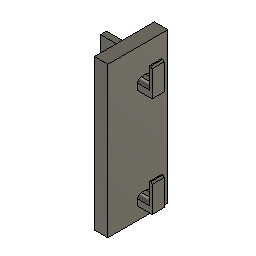
skadis_bracket_right (Autodesk Fusion 360 design; units mm, degrees)
part number: 2026-09-05-18-11-34-603
Autodesk Fusion 360 part; units mm, degrees
sketch "Plate" plane through (0, 0, 0) normal (0, 1, 0) x (1, 0, 0)
  line L0 (0, 0) -> (5.4, 0)
  line L1 (5.4, 0) -> (5.4, -60)
  line L2 (5.4, -60) -> (0, -60)
  line L3 (0, -60) -> (0, 0)
  dimension "d29" = 5.4
  dimension "d30" = 60
  constraint coincident L0.start L3.end
  constraint horizontal L0
  constraint horizontal L2
  constraint vertical L1
  constraint vertical L3
  measures "d29" horizontal distance of L0.start L1.end
  measures "d30" vertical distance of L0.start L1.end
extrude "Plate (1)" add sketch "Plate" along normal mid plane 24
sketch "Hook profile" plane through (0, 0, 0) normal (0, 1, 0) x (1, 0, 0)
  line L0 (0, -58) -> (-8.3, -58)
  line L1 (-8.3, -58) -> (-8.3, -41)
  line L2 (-8.3, -41) -> (-5.3, -41)
  line L3 (-5.3, -41) -> (-3.8, -42.5)
  line L4 (-3.8, -42.5) -> (-3.8, -53)
  line L5 (-3.8, -53) -> (0, -53)
  line L6 (0, -53) -> (0, -58)
  dimension "d33" = 58
  dimension "d34" = 8.3
  dimension "d35" = 3.8
  dimension "d36" = 5
  dimension "d37" = 10.5
  dimension "d38" = 1.5
  dimension "d39" = 1.5
  constraint horizontal L0
  constraint horizontal L2
  constraint horizontal L5
  constraint vertical L1
  constraint vertical L4
  constraint vertical L6
  constraint coincident origin L6
  measures "d33" vertical distance of origin L0.start
  measures "d34" horizontal distance of L0.start L0.end
  measures "d35" horizontal distance of L4.end L5.end
  measures "d36" vertical distance of L0.start L5.end
  measures "d37" vertical distance of L3.end L4.end
  measures "d38" horizontal distance of L2.end L3.end
  measures "d39" vertical distance of L2.end L3.end
extrude "Hook profile (1)" add sketch "Hook profile" along normal mid plane 2.4
pattern_linear "Hook rows" count 2 spacing 25.4 along (0, 0, -1) count 3 spacing 0 along (0, 0, 1) of "Hook profile (1)"
sketch "Peg profile" plane through (0, 0, 0) normal (0, 1, 0) x (1, 0, 0)
  line L0 (5.4, -45) -> (11.2, -45)
  line L1 (11.2, -45) -> (11.2, -55.4)
  line L2 (11.2, -55.4) -> (10.6, -56)
  line L3 (10.6, -56) -> (10.2, -56)
  line L4 (10.2, -56) -> (10.2, -49)
  line L5 (10.2, -49) -> (5.4, -49)
  line L6 (5.4, -49) -> (5.4, -45)
  dimension "d46" = 5.4
  dimension "d47" = 45
  dimension "d48" = 11.2
  dimension "d49" = 55.4
  dimension "d50" = 10.6
  dimension "d51" = 56
  dimension "d52" = 10.2
  dimension "d53" = 49
  constraint horizontal L0
  constraint horizontal L3
  constraint horizontal L5
  constraint vertical L1
  constraint vertical L4
  constraint vertical L6
  measures "d46" horizontal distance of origin L0.start
  measures "d47" vertical distance of origin L0.start
  measures "d48" horizontal distance of origin L0.end
  measures "d49" vertical distance of origin L1.end
  measures "d50" horizontal distance of origin L2.end
  measures "d51" vertical distance of origin L2.end
  measures "d52" horizontal distance of origin L3.end
  measures "d53" vertical distance of origin L4.end
extrude "Peg profile (1)" add sketch "Peg profile" along normal mid plane 4.8 from surface at 2.3
pattern_linear "Peg rows" count 2 spacing 40 along (0, 0, -1) count 3 spacing 0 along (0, 0, 1) of "Peg profile (1)"
fillet "Peg bearing fillets" radius 1.5 4 edges at (7.8, -0.1, 9) (7.8, 4.7, 9) (7.8, -0.1, 49) (7.8, 4.7, 49)
equation "bracketWidth = 24.0 mm" comment "bracket width across the upright"
equation "plateThickness = 5.4 mm" comment "board rear face sits on this"
equation "plateHeight = 60.0 mm" comment "plate height"
equation "slotWidth = 3.2 mm" comment "measured upright slot width"
equation "slotPitchVertical = 25.4 mm" comment "1 inch, measured"
equation "faceMetalThickness = 2.0 mm" comment "upright face metal"
equation "hookTabWidth = slotWidth - 0.8 mm" comment "blade width through the slot"
equation "hookThroat = faceMetalThickness + 1.8 mm" comment "gap behind the plate"
equation "hookNeckHeight = 5.0 mm" comment "bears on the slot bottom edge"
equation "hookLipThickness = 4.5 mm" comment "lip behind the upright face"
equation "hookLipDrop = 12.0 mm" comment "engagement below the neck"
equation "hookLipChamfer = 1.5 mm" comment "lead-in past slot burrs"
equation "topHookNeckTop = 58.0 mm" comment "top hook row"
equation "hookRows = 2" comment "hook rows (pattern count)"
equation "boardThickness = 4.6 mm" comment "SKADIS panel thickness"
equation "boardSlotWidth = 5.0 mm" comment "SKADIS slot width"
equation "boardSlotHeight = 15.0 mm" comment "SKADIS slot height"
equation "boardPitch = 40.0 mm" comment "SKADIS grid pitch"
equation "pegWidth = boardSlotWidth - 0.2 mm" comment "peg width in the slot"
equation "pegRootLength = boardThickness + 0.2 mm" comment "root through the board"
equation "pegRootHeight = 4.0 mm" comment "slot top edge bears on this"
equation "pegProngThickness = 1.0 mm" comment "prong in front of board"
equation "pegTotalHeight = boardSlotHeight - 4 mm" comment "prong rise above the root, and the lift needed to release"
equation "pegProngChamfer = 0.6 mm" comment "lead-in on the prong top"
equation "pegBearingFillet = 1.5 mm" comment "round on the root top edges the board bears on"
equation "topPegRootZ = 45.0 mm" comment "top peg root, above the plate foot"
equation "pegRows = 2" comment "pegs per bracket (pattern count)"
equation "pegOffsetY = 2.3 mm" comment "offset onto the board's 40 mm grid"
equation "d29 = plateThickness"
equation "d30 = plateHeight"
equation "d31 = bracketWidth"
equation "d33 = topHookNeckTop"
equation "d34 = hookThroat + hookLipThickness"
equation "d35 = hookThroat"
equation "d36 = hookNeckHeight"
equation "d37 = hookLipDrop - hookLipChamfer"
equation "d38 = hookLipChamfer"
equation "d39 = hookLipChamfer"
equation "d40 = hookTabWidth"
equation "d42 = hookRows"
equation "d44 = -slotPitchVertical"
equation "d46 = plateThickness"
equation "d47 = topPegRootZ"
equation "d48 = plateThickness + pegRootLength + pegProngThickness"
equation "d49 = topPegRootZ + pegTotalHeight - pegProngChamfer"
equation "d50 = plateThickness + pegRootLength + pegProngThickness - pegProngChamfer"
equation "d51 = topPegRootZ + pegTotalHeight"
equation "d52 = plateThickness + pegRootLength"
equation "d53 = topPegRootZ + pegRootHeight"
equation "d54 = pegOffsetY"
equation "d55 = pegWidth"
equation "d57 = pegRows"
equation "d59 = -boardPitch"
equation "d62 = pegBearingFillet"
named bodies: "skadis_bracket_right"
